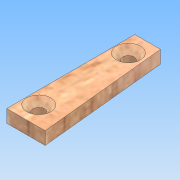
# Autodesk Inventor part: Pancake_Side Piece Short 3
Saved by Autodesk Inventor 2018.1 (Build 221171000, 171)
## iProperties
Created: 2019-02-22
Part Number: Pancake_Side Piece Short 3
Material: Wood (Birch)
Document SubType Name: Modeling
Designer: James
Density: 0.55 g/cm^3
Appearance: Birch - Natural Polished
Author: James
Autodesk Inventor part; units mm, degrees
ref_plane "YZ Plane" through (0, 0, 0) normal (1, 0, 0) x (0, 1, 0)
ref_plane "XZ Plane" through (0, 0, 0) normal (0, 1, 0) x (-1, 0, 0)
ref_plane "XY Plane" through (0, 0, 0) normal (0, 0, 1) x (1, 0, 0)
sketch "Sketch1" plane through (0, 0, 0) normal (0, 0, 1) x (1, 0, 0)
  line L0 (0, 0) -> (-15, 0)
  line L1 (-15, 0) -> (-15, 50)
  line L2 (-15, 50) -> (-5, 50)
  line L3 (-5, 50) -> (0, 0)
  dimension "d0" = 10
  dimension "d1" = 50
  dimension "d16" = 15
  constraints: 8 end point, 1 horizontal, 1 parallel, 1 perpendicular
  measures "d0" distance of L1.end L2.end
  measures "d1" distance of L0.end L1.end
  measures "d16" distance of L0.start L0.end
extrude "Extrusion1" add sketch "Sketch1" along normal blind 5
sketch "Sketch2" plane through (0, 0, 5) normal (0, 0, 1) x (1, 0, 0)
  line L0 (-15, 50) -> (-15, 0) projected
  line L1 (-5, 50) -> (-15, 50) projected
  line L2 (-15, 0) -> (0, 0) projected
  point P0 (-10, 42.5)
  point P1 (-10, 7.5)
  dimension "d6" = 7.5
  dimension "d7" = 7.5
  dimension "d8" = 35
  dimension "d17" = 5
  constraints: 1 vertical alignment
  measures "d6" distance from line of point (-10, 42.5) L1
  measures "d7" distance from line of L2 point (-10, 7.5)
  measures "d8" distance of point (-10, 42.5) point (-10, 7.5)
  measures "d17" distance from line of point (-10, 42.5) L0
hole "Hole1" at (-10, 42.5, 5) at (-10, 7.5, 5) direction (0, 0, -1) diameter 4.5 end through all countersink diameter 9.4 countersink angle 90 clearance for "Flat Head Machine Screw" size "M4" standard "Ansi Metric M Profile"
equation "\"d7\" = d6"
body "Solid1"
